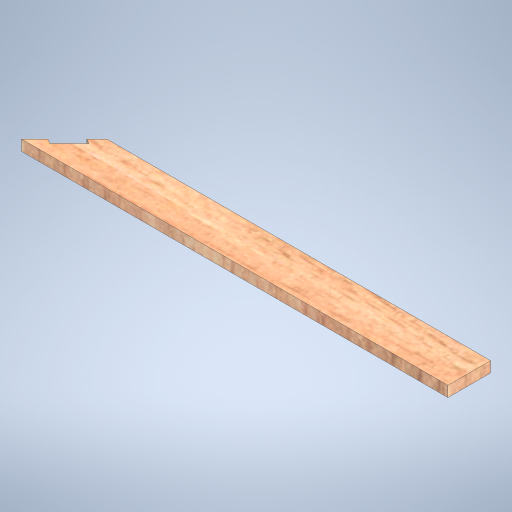
# Autodesk Inventor part: Yaxix
Saved by Autodesk Inventor 2023 (Build 270158000, 158)
## iProperties
Created: 2023-11-27
Part Number: Yaxix
Material: Wood (Birch)
Document SubType Name: Modeling
Designer: Mustapha
Density: 0.55 g/cm^3
Appearance: Birch - Natural Polished
Mass: 10.3617 g
Surface Area: 97.0307 cm^2
Volume: 18.8394 cm^3
Author: Mustapha
Autodesk Inventor part; units mm, degrees
ref_plane "YZ Plane" through (0, 0, 0) normal (1, 0, 0) x (0, 1, 0)
ref_plane "XZ Plane" through (0, 0, 0) normal (0, 1, 0) x (-1, 0, 0)
ref_plane "XY Plane" through (0, 0, 0) normal (0, 0, 1) x (1, 0, 0)
sketch "Sketch1" plane through (0, 0, 0) normal (0, 1, 0) x (-1, 0, 0)
  line L0 (0, 0) -> (200, 0)
  line L1 (200, 0) -> (200, -7.5533)
  line L2 (180, -20) -> (0, -20)
  line L3 (0, -20) -> (0, 0)
  line L4 (200, 0) -> (180, -20)
  line L5 (182.0213, -10) -> (194.6749, -10)
  line L6 (182.4568, -14.0077) -> (191.5424, -4.9221)
  line L7 (182.4568, -14.0077) -> (184.7026, -15.2974)
  line L8 (191.5424, -4.9221) -> (193.7882, -6.2118)
  point P0 (200, -10)
  dimension "d0" = 20
  dimension "d1" = 200
  dimension "d7" = 10
  dimension "d8" = 2.5
  dimension "d9" = 12.849
  constraints: 18 end point, 4 parallel, 3 point on line, 2 horizontal, 1 perpendicular
  measures "d0" distance between parallel lines of L0 L2
  measures "d1" distance of L0.start L0.end
  measures "d7" distance between parallel lines of L0 L5
  measures "d8" distance between parallel lines of L6 L4
  measures "d9" distance of L6.start L6.end
extrude "Extrusion1" add sketch "Sketch1" along normal blind 5 contours L0 L4 L8 L6 L7 L2 L3
body "Solid1"
